Autodesk Fusion 360 part; units mm, degrees
(part 3 of 5)
sketch "Sketch1 (2)" plane through (0, 0, 19.05) normal (0, 0, 1) x (-1, 0, 0) in component "spoilboard v12"
  line L0 (-99.06, -2093.1525) -> (-33.02, -2093.1525)
  arc A0 (-33.02, -2133.1525) -> (-33.02, -2093.1525) centre (-33.02, -2113.1525) ccw
  line L1 (-33.02, -2133.1525) -> (-99.06, -2133.1525)
  arc A1 (-99.06, -2093.1525) -> (-99.06, -2133.1525) centre (-99.06, -2113.1525) ccw
  arc A2 (-461.4333, -1693.1525) -> (-461.4333, -1733.1525) centre (-461.4333, -1713.1525) ccw
  line L2 (-461.4333, -1693.1525) -> (-395.3933, -1693.1525)
  arc A3 (-395.3933, -1733.1525) -> (-395.3933, -1693.1525) centre (-395.3933, -1713.1525) ccw
  line L3 (-395.3933, -1733.1525) -> (-461.4333, -1733.1525)
  line L4 (-99.06, -1913.1525) -> (-33.02, -1913.1525)
  arc A4 (-33.02, -1953.1525) -> (-33.02, -1913.1525) centre (-33.02, -1933.1525) ccw
  line L5 (-33.02, -1953.1525) -> (-99.06, -1953.1525)
  arc A5 (-99.06, -1913.1525) -> (-99.06, -1953.1525) centre (-99.06, -1933.1525) ccw
  line L6 (-99.06, -1293.1525) -> (-33.02, -1293.1525)
  arc A6 (-33.02, -1333.1525) -> (-33.02, -1293.1525) centre (-33.02, -1313.1525) ccw
  line L7 (-33.02, -1333.1525) -> (-99.06, -1333.1525)
  arc A7 (-99.06, -1293.1525) -> (-99.06, -1333.1525) centre (-99.06, -1313.1525) ccw
  arc A8 (-642.62, -2093.1525) -> (-642.62, -2133.1525) centre (-642.62, -2113.1525) ccw
  line L8 (-642.62, -2093.1525) -> (-576.58, -2093.1525)
  arc A9 (-576.58, -2133.1525) -> (-576.58, -2093.1525) centre (-576.58, -2113.1525) ccw
  line L9 (-576.58, -2133.1525) -> (-642.62, -2133.1525)
  arc A10 (-642.62, -2313.1525) -> (-642.62, -2353.1525) centre (-642.62, -2333.1525) ccw
  line L10 (-642.62, -2313.1525) -> (-576.58, -2313.1525)
  arc A11 (-576.58, -2353.1525) -> (-576.58, -2313.1525) centre (-576.58, -2333.1525) ccw
  line L11 (-576.58, -2353.1525) -> (-642.62, -2353.1525)
  arc A12 (-642.62, -1693.1525) -> (-642.62, -1733.1525) centre (-642.62, -1713.1525) ccw
  line L12 (-642.62, -1693.1525) -> (-576.58, -1693.1525)
  arc A13 (-576.58, -1733.1525) -> (-576.58, -1693.1525) centre (-576.58, -1713.1525) ccw
  line L13 (-576.58, -1733.1525) -> (-642.62, -1733.1525)
  arc A14 (-642.62, -1913.1525) -> (-642.62, -1953.1525) centre (-642.62, -1933.1525) ccw
  line L14 (-642.62, -1913.1525) -> (-576.58, -1913.1525)
  arc A15 (-576.58, -1953.1525) -> (-576.58, -1913.1525) centre (-576.58, -1933.1525) ccw
  line L15 (-576.58, -1953.1525) -> (-642.62, -1953.1525)
  arc A16 (-642.62, -1293.1525) -> (-642.62, -1333.1525) centre (-642.62, -1313.1525) ccw
  line L16 (-642.62, -1293.1525) -> (-576.58, -1293.1525)
  arc A17 (-576.58, -1333.1525) -> (-576.58, -1293.1525) centre (-576.58, -1313.1525) ccw
  line L17 (-576.58, -1333.1525) -> (-642.62, -1333.1525)
  arc A18 (-642.62, -1513.1525) -> (-642.62, -1553.1525) centre (-642.62, -1533.1525) ccw
  line L18 (-642.62, -1513.1525) -> (-576.58, -1513.1525)
  arc A19 (-576.58, -1553.1525) -> (-576.58, -1513.1525) centre (-576.58, -1533.1525) ccw
  line L19 (-576.58, -1553.1525) -> (-642.62, -1553.1525)
  line L20 (-33.02, -133.1525) -> (-99.06, -133.1525)
  arc A20 (-99.06, -93.1525) -> (-99.06, -133.1525) centre (-99.06, -113.1525) ccw
  line L21 (-99.06, -93.1525) -> (-33.02, -93.1525)
  arc A21 (-33.02, -133.1525) -> (-33.02, -93.1525) centre (-33.02, -113.1525) ccw
  line L22 (-214.2067, -353.1525) -> (-280.2467, -353.1525)
  arc A22 (-280.2467, -313.1525) -> (-280.2467, -353.1525) centre (-280.2467, -333.1525) ccw
  line L23 (-280.2467, -313.1525) -> (-214.2067, -313.1525)
  arc A23 (-214.2067, -353.1525) -> (-214.2067, -313.1525) centre (-214.2067, -333.1525) ccw
  arc A24 (-461.4333, -713.1525) -> (-461.4333, -753.1525) centre (-461.4333, -733.1525) ccw
  line L24 (-461.4333, -713.1525) -> (-395.3933, -713.1525)
  arc A25 (-395.3933, -753.1525) -> (-395.3933, -713.1525) centre (-395.3933, -733.1525) ccw
  line L25 (-395.3933, -753.1525) -> (-461.4333, -753.1525)
  arc A26 (-280.2467, -1113.1525) -> (-280.2467, -1153.1525) centre (-280.2467, -1133.1525) ccw
  line L26 (-280.2467, -1113.1525) -> (-214.2067, -1113.1525)
  arc A27 (-214.2067, -1153.1525) -> (-214.2067, -1113.1525) centre (-214.2067, -1133.1525) ccw
  line L27 (-214.2067, -1153.1525) -> (-280.2467, -1153.1525)
  line L28 (-280.2467, -893.1525) -> (-214.2067, -893.1525)
  arc A28 (-214.2067, -933.1525) -> (-214.2067, -893.1525) centre (-214.2067, -913.1525) ccw
  line L29 (-214.2067, -933.1525) -> (-280.2467, -933.1525)
  arc A29 (-280.2467, -893.1525) -> (-280.2467, -933.1525) centre (-280.2467, -913.1525) ccw
  line L30 (-1120.14, -133.1525) -> (-1186.18, -133.1525)
  arc A30 (-1186.18, -93.1525) -> (-1186.18, -133.1525) centre (-1186.18, -113.1525) ccw
  line L31 (-1186.18, -93.1525) -> (-1120.14, -93.1525)
  arc A31 (-1120.14, -133.1525) -> (-1120.14, -93.1525) centre (-1120.14, -113.1525) ccw
  line L32 (-1120.14, -353.1525) -> (-1186.18, -353.1525)
  arc A32 (-1186.18, -313.1525) -> (-1186.18, -353.1525) centre (-1186.18, -333.1525) ccw
  line L33 (-1186.18, -313.1525) -> (-1120.14, -313.1525)
  arc A33 (-1120.14, -353.1525) -> (-1120.14, -313.1525) centre (-1120.14, -333.1525) ccw
  arc A34 (-642.62, -713.1525) -> (-642.62, -753.1525) centre (-642.62, -733.1525) ccw
  line L34 (-642.62, -713.1525) -> (-576.58, -713.1525)
  arc A35 (-576.58, -753.1525) -> (-576.58, -713.1525) centre (-576.58, -733.1525) ccw
  line L35 (-576.58, -753.1525) -> (-642.62, -753.1525)
  arc A36 (-642.62, -493.1525) -> (-642.62, -533.1525) centre (-642.62, -513.1525) ccw
  line L36 (-642.62, -493.1525) -> (-576.58, -493.1525)
  arc A37 (-576.58, -533.1525) -> (-576.58, -493.1525) centre (-576.58, -513.1525) ccw
  line L37 (-576.58, -533.1525) -> (-642.62, -533.1525)
  arc A38 (-642.62, -1113.1525) -> (-642.62, -1153.1525) centre (-642.62, -1133.1525) ccw
  line L38 (-642.62, -1113.1525) -> (-576.58, -1113.1525)
  arc A39 (-576.58, -1153.1525) -> (-576.58, -1113.1525) centre (-576.58, -1133.1525) ccw
  line L39 (-576.58, -1153.1525) -> (-642.62, -1153.1525)
  arc A40 (-642.62, -893.1525) -> (-642.62, -933.1525) centre (-642.62, -913.1525) ccw
  line L40 (-642.62, -893.1525) -> (-576.58, -893.1525)
  arc A41 (-576.58, -933.1525) -> (-576.58, -893.1525) centre (-576.58, -913.1525) ccw
  line L41 (-576.58, -933.1525) -> (-642.62, -933.1525)
  line L42 (-757.7667, -933.1525) -> (-823.8067, -933.1525)
  arc A42 (-823.8067, -893.1525) -> (-823.8067, -933.1525) centre (-823.8067, -913.1525) ccw
  line L43 (-823.8067, -893.1525) -> (-757.7667, -893.1525)
  arc A43 (-757.7667, -933.1525) -> (-757.7667, -893.1525) centre (-757.7667, -913.1525) ccw
  line L44 (-757.7667, -1153.1525) -> (-823.8067, -1153.1525)
  arc A44 (-823.8067, -1113.1525) -> (-823.8067, -1153.1525) centre (-823.8067, -1133.1525) ccw
  line L45 (-823.8067, -1113.1525) -> (-757.7667, -1113.1525)
  arc A45 (-757.7667, -1153.1525) -> (-757.7667, -1113.1525) centre (-757.7667, -1133.1525) ccw
  line L46 (-757.7667, -533.1525) -> (-823.8067, -533.1525)
  arc A46 (-823.8067, -493.1525) -> (-823.8067, -533.1525) centre (-823.8067, -513.1525) ccw
  line L47 (-823.8067, -493.1525) -> (-757.7667, -493.1525)
  arc A47 (-757.7667, -533.1525) -> (-757.7667, -493.1525) centre (-757.7667, -513.1525) ccw
  line L48 (-757.7667, -753.1525) -> (-823.8067, -753.1525)
  arc A48 (-823.8067, -713.1525) -> (-823.8067, -753.1525) centre (-823.8067, -733.1525) ccw
  line L49 (-823.8067, -713.1525) -> (-757.7667, -713.1525)
  arc A49 (-757.7667, -753.1525) -> (-757.7667, -713.1525) centre (-757.7667, -733.1525) ccw
  line L50 (-938.9533, -353.1525) -> (-1004.9933, -353.1525)
  arc A50 (-1004.9933, -313.1525) -> (-1004.9933, -353.1525) centre (-1004.9933, -333.1525) ccw
  line L51 (-1004.9933, -313.1525) -> (-938.9533, -313.1525)
  arc A51 (-938.9533, -353.1525) -> (-938.9533, -313.1525) centre (-938.9533, -333.1525) ccw
  line L52 (-938.9533, -133.1525) -> (-1004.9933, -133.1525)
  arc A52 (-1004.9933, -93.1525) -> (-1004.9933, -133.1525) centre (-1004.9933, -113.1525) ccw
  line L53 (-1004.9933, -93.1525) -> (-938.9533, -93.1525)
  arc A53 (-938.9533, -133.1525) -> (-938.9533, -93.1525) centre (-938.9533, -113.1525) ccw
  line L54 (-99.06, -893.1525) -> (-33.02, -893.1525)
  arc A54 (-33.02, -933.1525) -> (-33.02, -893.1525) centre (-33.02, -913.1525) ccw
  line L55 (-33.02, -933.1525) -> (-99.06, -933.1525)
  arc A55 (-99.06, -893.1525) -> (-99.06, -933.1525) centre (-99.06, -913.1525) ccw
  arc A56 (-461.4333, -493.1525) -> (-461.4333, -533.1525) centre (-461.4333, -513.1525) ccw
  line L56 (-461.4333, -493.1525) -> (-395.3933, -493.1525)
  arc A57 (-395.3933, -533.1525) -> (-395.3933, -493.1525) centre (-395.3933, -513.1525) ccw
  line L57 (-395.3933, -533.1525) -> (-461.4333, -533.1525)
  line L58 (-99.06, -713.1525) -> (-33.02, -713.1525)
  arc A58 (-33.02, -753.1525) -> (-33.02, -713.1525) centre (-33.02, -733.1525) ccw
  line L59 (-33.02, -753.1525) -> (-99.06, -753.1525)
  arc A59 (-99.06, -713.1525) -> (-99.06, -753.1525) centre (-99.06, -733.1525) ccw
  line L60 (-33.02, -353.1525) -> (-99.06, -353.1525)
  arc A60 (-99.06, -313.1525) -> (-99.06, -353.1525) centre (-99.06, -333.1525) ccw
  line L61 (-99.06, -313.1525) -> (-33.02, -313.1525)
  arc A61 (-33.02, -353.1525) -> (-33.02, -313.1525) centre (-33.02, -333.1525) ccw
  line L62 (-1186.18, -1513.1525) -> (-1120.14, -1513.1525)
  arc A62 (-1120.14, -1553.1525) -> (-1120.14, -1513.1525) centre (-1120.14, -1533.1525) ccw
  line L63 (-1120.14, -1553.1525) -> (-1186.18, -1553.1525)
  arc A63 (-1186.18, -1513.1525) -> (-1186.18, -1553.1525) centre (-1186.18, -1533.1525) ccw
  line L64 (-1120.14, -1333.1525) -> (-1186.18, -1333.1525)
  arc A64 (-1186.18, -1293.1525) -> (-1186.18, -1333.1525) centre (-1186.18, -1313.1525) ccw
  line L65 (-1186.18, -1293.1525) -> (-1120.14, -1293.1525)
  arc A65 (-1120.14, -1333.1525) -> (-1120.14, -1293.1525) centre (-1120.14, -1313.1525) ccw
  line L66 (-1186.18, -1913.1525) -> (-1120.14, -1913.1525)
  arc A66 (-1120.14, -1953.1525) -> (-1120.14, -1913.1525) centre (-1120.14, -1933.1525) ccw
  line L67 (-1120.14, -1953.1525) -> (-1186.18, -1953.1525)
  arc A67 (-1186.18, -1913.1525) -> (-1186.18, -1953.1525) centre (-1186.18, -1933.1525) ccw
  line L68 (-1120.14, -1733.1525) -> (-1186.18, -1733.1525)
  arc A68 (-1186.18, -1693.1525) -> (-1186.18, -1733.1525) centre (-1186.18, -1713.1525) ccw
  line L69 (-1186.18, -1693.1525) -> (-1120.14, -1693.1525)
  arc A69 (-1120.14, -1733.1525) -> (-1120.14, -1693.1525) centre (-1120.14, -1713.1525) ccw
  line L70 (-1186.18, -2313.1525) -> (-1120.14, -2313.1525)
  arc A70 (-1120.14, -2353.1525) -> (-1120.14, -2313.1525) centre (-1120.14, -2333.1525) ccw
  line L71 (-1120.14, -2353.1525) -> (-1186.18, -2353.1525)
  arc A71 (-1186.18, -2313.1525) -> (-1186.18, -2353.1525) centre (-1186.18, -2333.1525) ccw
  line L72 (-1120.14, -2133.1525) -> (-1186.18, -2133.1525)
  arc A72 (-1186.18, -2093.1525) -> (-1186.18, -2133.1525) centre (-1186.18, -2113.1525) ccw
  line L73 (-1186.18, -2093.1525) -> (-1120.14, -2093.1525)
  arc A73 (-1120.14, -2133.1525) -> (-1120.14, -2093.1525) centre (-1120.14, -2113.1525) ccw
  arc A74 (-280.2467, -1513.1525) -> (-280.2467, -1553.1525) centre (-280.2467, -1533.1525) ccw
  line L74 (-280.2467, -1513.1525) -> (-214.2067, -1513.1525)
  arc A75 (-214.2067, -1553.1525) -> (-214.2067, -1513.1525) centre (-214.2067, -1533.1525) ccw
  line L75 (-214.2067, -1553.1525) -> (-280.2467, -1553.1525)
  line L76 (-280.2467, -1293.1525) -> (-214.2067, -1293.1525)
  arc A76 (-214.2067, -1333.1525) -> (-214.2067, -1293.1525) centre (-214.2067, -1313.1525) ccw
  line L77 (-214.2067, -1333.1525) -> (-280.2467, -1333.1525)
  arc A77 (-280.2467, -1293.1525) -> (-280.2467, -1333.1525) centre (-280.2467, -1313.1525) ccw
  arc A78 (-461.4333, -1913.1525) -> (-461.4333, -1953.1525) centre (-461.4333, -1933.1525) ccw
  line L78 (-461.4333, -1913.1525) -> (-395.3933, -1913.1525)
  arc A79 (-395.3933, -1953.1525) -> (-395.3933, -1913.1525) centre (-395.3933, -1933.1525) ccw
  line L79 (-395.3933, -1953.1525) -> (-461.4333, -1953.1525)
  arc A80 (-280.2467, -2313.1525) -> (-280.2467, -2353.1525) centre (-280.2467, -2333.1525) ccw
  line L80 (-280.2467, -2313.1525) -> (-214.2067, -2313.1525)
  arc A81 (-214.2067, -2353.1525) -> (-214.2067, -2313.1525) centre (-214.2067, -2333.1525) ccw
  line L81 (-214.2067, -2353.1525) -> (-280.2467, -2353.1525)
  line L82 (-280.2467, -2093.1525) -> (-214.2067, -2093.1525)
  arc A82 (-214.2067, -2133.1525) -> (-214.2067, -2093.1525) centre (-214.2067, -2113.1525) ccw
  line L83 (-214.2067, -2133.1525) -> (-280.2467, -2133.1525)
  arc A83 (-280.2467, -2093.1525) -> (-280.2467, -2133.1525) centre (-280.2467, -2113.1525) ccw
  arc A84 (-461.4333, -2313.1525) -> (-461.4333, -2353.1525) centre (-461.4333, -2333.1525) ccw
  line L84 (-461.4333, -2313.1525) -> (-395.3933, -2313.1525)
  arc A85 (-395.3933, -2353.1525) -> (-395.3933, -2313.1525) centre (-395.3933, -2333.1525) ccw
  line L85 (-395.3933, -2353.1525) -> (-461.4333, -2353.1525)
  line L86 (-280.2467, -1693.1525) -> (-214.2067, -1693.1525)
  arc A86 (-214.2067, -1733.1525) -> (-214.2067, -1693.1525) centre (-214.2067, -1713.1525) ccw
  line L87 (-214.2067, -1733.1525) -> (-280.2467, -1733.1525)
  arc A87 (-280.2467, -1693.1525) -> (-280.2467, -1733.1525) centre (-280.2467, -1713.1525) ccw
  arc A88 (-280.2467, -1913.1525) -> (-280.2467, -1953.1525) centre (-280.2467, -1933.1525) ccw
  line L88 (-280.2467, -1913.1525) -> (-214.2067, -1913.1525)
  arc A89 (-214.2067, -1953.1525) -> (-214.2067, -1913.1525) centre (-214.2067, -1933.1525) ccw
  line L89 (-214.2067, -1953.1525) -> (-280.2467, -1953.1525)
  arc A90 (-461.4333, -1513.1525) -> (-461.4333, -1553.1525) centre (-461.4333, -1533.1525) ccw
  line L90 (-461.4333, -1513.1525) -> (-395.3933, -1513.1525)
  arc A91 (-395.3933, -1553.1525) -> (-395.3933, -1513.1525) centre (-395.3933, -1533.1525) ccw
  line L91 (-395.3933, -1553.1525) -> (-461.4333, -1553.1525)
  line L92 (-757.7667, -2133.1525) -> (-823.8067, -2133.1525)
  arc A92 (-823.8067, -2093.1525) -> (-823.8067, -2133.1525) centre (-823.8067, -2113.1525) ccw
  line L93 (-823.8067, -2093.1525) -> (-757.7667, -2093.1525)
  arc A93 (-757.7667, -2133.1525) -> (-757.7667, -2093.1525) centre (-757.7667, -2113.1525) ccw
  line L94 (-757.7667, -2353.1525) -> (-823.8067, -2353.1525)
  arc A94 (-823.8067, -2313.1525) -> (-823.8067, -2353.1525) centre (-823.8067, -2333.1525) ccw
  line L95 (-823.8067, -2313.1525) -> (-757.7667, -2313.1525)
  arc A95 (-757.7667, -2353.1525) -> (-757.7667, -2313.1525) centre (-757.7667, -2333.1525) ccw
  line L96 (-757.7667, -1733.1525) -> (-823.8067, -1733.1525)
  arc A96 (-823.8067, -1693.1525) -> (-823.8067, -1733.1525) centre (-823.8067, -1713.1525) ccw
  line L97 (-823.8067, -1693.1525) -> (-757.7667, -1693.1525)
  arc A97 (-757.7667, -1733.1525) -> (-757.7667, -1693.1525) centre (-757.7667, -1713.1525) ccw
  line L98 (-757.7667, -1953.1525) -> (-823.8067, -1953.1525)
  arc A98 (-823.8067, -1913.1525) -> (-823.8067, -1953.1525) centre (-823.8067, -1933.1525) ccw
  line L99 (-823.8067, -1913.1525) -> (-757.7667, -1913.1525)
  arc A99 (-757.7667, -1953.1525) -> (-757.7667, -1913.1525) centre (-757.7667, -1933.1525) ccw
  line L100 (-757.7667, -1333.1525) -> (-823.8067, -1333.1525)
  arc A100 (-823.8067, -1293.1525) -> (-823.8067, -1333.1525) centre (-823.8067, -1313.1525) ccw
  line L101 (-823.8067, -1293.1525) -> (-757.7667, -1293.1525)
  arc A101 (-757.7667, -1333.1525) -> (-757.7667, -1293.1525) centre (-757.7667, -1313.1525) ccw
  line L102 (-757.7667, -1553.1525) -> (-823.8067, -1553.1525)
  arc A102 (-823.8067, -1513.1525) -> (-823.8067, -1553.1525) centre (-823.8067, -1533.1525) ccw
  line L103 (-823.8067, -1513.1525) -> (-757.7667, -1513.1525)
  arc A103 (-757.7667, -1553.1525) -> (-757.7667, -1513.1525) centre (-757.7667, -1533.1525) ccw
  line L104 (-214.2067, -133.1525) -> (-280.2467, -133.1525)
  arc A104 (-280.2467, -93.1525) -> (-280.2467, -133.1525) centre (-280.2467, -113.1525) ccw
  line L105 (-280.2467, -93.1525) -> (-214.2067, -93.1525)
  arc A105 (-214.2067, -133.1525) -> (-214.2067, -93.1525) centre (-214.2067, -113.1525) ccw
  line L106 (-395.3933, -353.1525) -> (-461.4333, -353.1525)
  arc A106 (-461.4333, -313.1525) -> (-461.4333, -353.1525) centre (-461.4333, -333.1525) ccw
  line L107 (-461.4333, -313.1525) -> (-395.3933, -313.1525)
  arc A107 (-395.3933, -353.1525) -> (-395.3933, -313.1525) centre (-395.3933, -333.1525) ccw
  line L108 (-99.06, -493.1525) -> (-33.02, -493.1525)
  arc A108 (-33.02, -533.1525) -> (-33.02, -493.1525) centre (-33.02, -513.1525) ccw
  line L109 (-33.02, -533.1525) -> (-99.06, -533.1525)
  arc A109 (-99.06, -493.1525) -> (-99.06, -533.1525) centre (-99.06, -513.1525) ccw
  line L110 (-99.06, -1113.1525) -> (-33.02, -1113.1525)
  arc A110 (-33.02, -1153.1525) -> (-33.02, -1113.1525) centre (-33.02, -1133.1525) ccw
  line L111 (-33.02, -1153.1525) -> (-99.06, -1153.1525)
  arc A111 (-99.06, -1113.1525) -> (-99.06, -1153.1525) centre (-99.06, -1133.1525) ccw
  arc A112 (-461.4333, -893.1525) -> (-461.4333, -933.1525) centre (-461.4333, -913.1525) ccw
  line L112 (-461.4333, -893.1525) -> (-395.3933, -893.1525)
  arc A113 (-395.3933, -933.1525) -> (-395.3933, -893.1525) centre (-395.3933, -913.1525) ccw
  line L113 (-395.3933, -933.1525) -> (-461.4333, -933.1525)
  line L114 (-576.58, -353.1525) -> (-642.62, -353.1525)
  arc A114 (-642.62, -313.1525) -> (-642.62, -353.1525) centre (-642.62, -333.1525) ccw
  line L115 (-642.62, -313.1525) -> (-576.58, -313.1525)
  arc A115 (-576.58, -353.1525) -> (-576.58, -313.1525) centre (-576.58, -333.1525) ccw
  line L116 (-1186.18, -713.1525) -> (-1120.14, -713.1525)
  arc A116 (-1120.14, -753.1525) -> (-1120.14, -713.1525) centre (-1120.14, -733.1525) ccw
  line L117 (-1120.14, -753.1525) -> (-1186.18, -753.1525)
  arc A117 (-1186.18, -713.1525) -> (-1186.18, -753.1525) centre (-1186.18, -733.1525) ccw
  line L118 (-1120.14, -533.1525) -> (-1186.18, -533.1525)
  arc A118 (-1186.18, -493.1525) -> (-1186.18, -533.1525) centre (-1186.18, -513.1525) ccw
  line L119 (-1186.18, -493.1525) -> (-1120.14, -493.1525)
  arc A119 (-1120.14, -533.1525) -> (-1120.14, -493.1525) centre (-1120.14, -513.1525) ccw
  line L120 (-1186.18, -1113.1525) -> (-1120.14, -1113.1525)
  arc A120 (-1120.14, -1153.1525) -> (-1120.14, -1113.1525) centre (-1120.14, -1133.1525) ccw
  line L121 (-1120.14, -1153.1525) -> (-1186.18, -1153.1525)
  arc A121 (-1186.18, -1113.1525) -> (-1186.18, -1153.1525) centre (-1186.18, -1133.1525) ccw
  line L122 (-1120.14, -933.1525) -> (-1186.18, -933.1525)
  arc A122 (-1186.18, -893.1525) -> (-1186.18, -933.1525) centre (-1186.18, -913.1525) ccw
  line L123 (-1186.18, -893.1525) -> (-1120.14, -893.1525)
  arc A123 (-1120.14, -933.1525) -> (-1120.14, -893.1525) centre (-1120.14, -913.1525) ccw
  line L124 (-576.58, -133.1525) -> (-642.62, -133.1525)
  arc A124 (-642.62, -93.1525) -> (-642.62, -133.1525) centre (-642.62, -113.1525) ccw
  line L125 (-642.62, -93.1525) -> (-576.58, -93.1525)
  arc A125 (-576.58, -133.1525) -> (-576.58, -93.1525) centre (-576.58, -113.1525) ccw
  line L126 (-938.9533, -933.1525) -> (-1004.9933, -933.1525)
  arc A126 (-1004.9933, -893.1525) -> (-1004.9933, -933.1525) centre (-1004.9933, -913.1525) ccw
  line L127 (-1004.9933, -893.1525) -> (-938.9533, -893.1525)
  arc A127 (-938.9533, -933.1525) -> (-938.9533, -893.1525) centre (-938.9533, -913.1525) ccw
  arc A128 (-1004.9933, -1113.1525) -> (-1004.9933, -1153.1525) centre (-1004.9933, -1133.1525) ccw
  line L128 (-1004.9933, -1113.1525) -> (-938.9533, -1113.1525)
  arc A129 (-938.9533, -1153.1525) -> (-938.9533, -1113.1525) centre (-938.9533, -1133.1525) ccw
  line L129 (-938.9533, -1153.1525) -> (-1004.9933, -1153.1525)
  line L130 (-938.9533, -533.1525) -> (-1004.9933, -533.1525)
  arc A130 (-1004.9933, -493.1525) -> (-1004.9933, -533.1525) centre (-1004.9933, -513.1525) ccw
  line L131 (-1004.9933, -493.1525) -> (-938.9533, -493.1525)
  arc A131 (-938.9533, -533.1525) -> (-938.9533, -493.1525) centre (-938.9533, -513.1525) ccw
  arc A132 (-1004.9933, -713.1525) -> (-1004.9933, -753.1525) centre (-1004.9933, -733.1525) ccw
  line L132 (-1004.9933, -713.1525) -> (-938.9533, -713.1525)
  arc A133 (-938.9533, -753.1525) -> (-938.9533, -713.1525) centre (-938.9533, -733.1525) ccw
  line L133 (-938.9533, -753.1525) -> (-1004.9933, -753.1525)
  line L134 (-757.7667, -353.1525) -> (-823.8067, -353.1525)
  arc A134 (-823.8067, -313.1525) -> (-823.8067, -353.1525) centre (-823.8067, -333.1525) ccw
  line L135 (-823.8067, -313.1525) -> (-757.7667, -313.1525)
  arc A135 (-757.7667, -353.1525) -> (-757.7667, -313.1525) centre (-757.7667, -333.1525) ccw
  line L136 (-757.7667, -133.1525) -> (-823.8067, -133.1525)
  arc A136 (-823.8067, -93.1525) -> (-823.8067, -133.1525) centre (-823.8067, -113.1525) ccw
  line L137 (-823.8067, -93.1525) -> (-757.7667, -93.1525)
  arc A137 (-757.7667, -133.1525) -> (-757.7667, -93.1525) centre (-757.7667, -113.1525) ccw
  arc A138 (-461.4333, -1113.1525) -> (-461.4333, -1153.1525) centre (-461.4333, -1133.1525) ccw
  line L138 (-461.4333, -1113.1525) -> (-395.3933, -1113.1525)
  arc A139 (-395.3933, -1153.1525) -> (-395.3933, -1113.1525) centre (-395.3933, -1133.1525) ccw
  line L139 (-395.3933, -1153.1525) -> (-461.4333, -1153.1525)
  line L140 (-280.2467, -493.1525) -> (-214.2067, -493.1525)
  arc A140 (-214.2067, -533.1525) -> (-214.2067, -493.1525) centre (-214.2067, -513.1525) ccw
  line L141 (-214.2067, -533.1525) -> (-280.2467, -533.1525)
  arc A141 (-280.2467, -493.1525) -> (-280.2467, -533.1525) centre (-280.2467, -513.1525) ccw
  arc A142 (-280.2467, -713.1525) -> (-280.2467, -753.1525) centre (-280.2467, -733.1525) ccw
  line L142 (-280.2467, -713.1525) -> (-214.2067, -713.1525)
  arc A143 (-214.2067, -753.1525) -> (-214.2067, -713.1525) centre (-214.2067, -733.1525) ccw
  line L143 (-214.2067, -753.1525) -> (-280.2467, -753.1525)
  line L144 (-395.3933, -133.1525) -> (-461.4333, -133.1525)
  arc A144 (-461.4333, -93.1525) -> (-461.4333, -133.1525) centre (-461.4333, -113.1525) ccw
  line L145 (-461.4333, -93.1525) -> (-395.3933, -93.1525)
  arc A145 (-395.3933, -133.1525) -> (-395.3933, -93.1525) centre (-395.3933, -113.1525) ccw
  arc A146 (-1004.9933, -1513.1525) -> (-1004.9933, -1553.1525) centre (-1004.9933, -1533.1525) ccw
  line L146 (-1004.9933, -1513.1525) -> (-938.9533, -1513.1525)
  arc A147 (-938.9533, -1553.1525) -> (-938.9533, -1513.1525) centre (-938.9533, -1533.1525) ccw
  line L147 (-938.9533, -1553.1525) -> (-1004.9933, -1553.1525)
  line L148 (-938.9533, -1333.1525) -> (-1004.9933, -1333.1525)
  arc A148 (-1004.9933, -1293.1525) -> (-1004.9933, -1333.1525) centre (-1004.9933, -1313.1525) ccw
  line L149 (-1004.9933, -1293.1525) -> (-938.9533, -1293.1525)
  arc A149 (-938.9533, -1333.1525) -> (-938.9533, -1293.1525) centre (-938.9533, -1313.1525) ccw
  arc A150 (-1004.9933, -1913.1525) -> (-1004.9933, -1953.1525) centre (-1004.9933, -1933.1525) ccw
  line L150 (-1004.9933, -1913.1525) -> (-938.9533, -1913.1525)
  arc A151 (-938.9533, -1953.1525) -> (-938.9533, -1913.1525) centre (-938.9533, -1933.1525) ccw
  line L151 (-938.9533, -1953.1525) -> (-1004.9933, -1953.1525)
  line L152 (-938.9533, -1733.1525) -> (-1004.9933, -1733.1525)
  arc A152 (-1004.9933, -1693.1525) -> (-1004.9933, -1733.1525) centre (-1004.9933, -1713.1525) ccw
  line L153 (-1004.9933, -1693.1525) -> (-938.9533, -1693.1525)
  arc A153 (-938.9533, -1733.1525) -> (-938.9533, -1693.1525) centre (-938.9533, -1713.1525) ccw
  arc A154 (-1004.9933, -2313.1525) -> (-1004.9933, -2353.1525) centre (-1004.9933, -2333.1525) ccw
  line L154 (-1004.9933, -2313.1525) -> (-938.9533, -2313.1525)
  arc A155 (-938.9533, -2353.1525) -> (-938.9533, -2313.1525) centre (-938.9533, -2333.1525) ccw
  line L155 (-938.9533, -2353.1525) -> (-1004.9933, -2353.1525)
  line L156 (-938.9533, -2133.1525) -> (-1004.9933, -2133.1525)
  arc A156 (-1004.9933, -2093.1525) -> (-1004.9933, -2133.1525) centre (-1004.9933, -2113.1525) ccw
  line L157 (-1004.9933, -2093.1525) -> (-938.9533, -2093.1525)
  arc A157 (-938.9533, -2133.1525) -> (-938.9533, -2093.1525) centre (-938.9533, -2113.1525) ccw
  line L158 (-99.06, -1513.1525) -> (-33.02, -1513.1525)
  arc A158 (-33.02, -1553.1525) -> (-33.02, -1513.1525) centre (-33.02, -1533.1525) ccw
  line L159 (-33.02, -1553.1525) -> (-99.06, -1553.1525)
  arc A159 (-99.06, -1513.1525) -> (-99.06, -1553.1525) centre (-99.06, -1533.1525) ccw
  arc A160 (-461.4333, -1293.1525) -> (-461.4333, -1333.1525) centre (-461.4333, -1313.1525) ccw
  line L160 (-461.4333, -1293.1525) -> (-395.3933, -1293.1525)
  arc A161 (-395.3933, -1333.1525) -> (-395.3933, -1293.1525) centre (-395.3933, -1313.1525) ccw
  line L161 (-395.3933, -1333.1525) -> (-461.4333, -1333.1525)
  line L162 (-99.06, -1693.1525) -> (-33.02, -1693.1525)
  arc A162 (-33.02, -1733.1525) -> (-33.02, -1693.1525) centre (-33.02, -1713.1525) ccw
  line L163 (-33.02, -1733.1525) -> (-99.06, -1733.1525)
  arc A163 (-99.06, -1693.1525) -> (-99.06, -1733.1525) centre (-99.06, -1713.1525) ccw
  line L164 (-99.06, -2313.1525) -> (-33.02, -2313.1525)
  arc A164 (-33.02, -2353.1525) -> (-33.02, -2313.1525) centre (-33.02, -2333.1525) ccw
  line L165 (-33.02, -2353.1525) -> (-99.06, -2353.1525)
  arc A165 (-99.06, -2313.1525) -> (-99.06, -2353.1525) centre (-99.06, -2333.1525) ccw
  arc A166 (-461.4333, -2093.1525) -> (-461.4333, -2133.1525) centre (-461.4333, -2113.1525) ccw
  line L166 (-461.4333, -2093.1525) -> (-395.3933, -2093.1525)
  arc A167 (-395.3933, -2133.1525) -> (-395.3933, -2093.1525) centre (-395.3933, -2113.1525) ccw
  line L167 (-395.3933, -2133.1525) -> (-461.4333, -2133.1525)
  circle A168 centre (-34.29, -2020) radius 17.145
  circle A169 centre (-321.945, -2020) radius 17.145
  circle A170 centre (-609.6, -2020) radius 17.145
  circle A171 centre (-321.945, -420) radius 17.145
  circle A172 centre (-897.255, -2020) radius 17.145
  circle A173 centre (-1184.91, -2020) radius 17.145
  circle A174 centre (-34.29, -420) radius 17.145
  circle A175 centre (-34.29, -2420) radius 17.145
  circle A176 centre (-1184.91, -20) radius 17.145
  circle A177 centre (-321.945, -2420) radius 17.145
  circle A178 centre (-609.6, -2420) radius 17.145
  circle A179 centre (-897.255, -20) radius 17.145
  circle A180 centre (-897.255, -2420) radius 17.145
  circle A181 centre (-321.945, -1220) radius 17.145
  circle A182 centre (-34.29, -1220) radius 17.145
  circle A183 centre (-1184.91, -820) radius 17.145
  circle A184 centre (-897.255, -820) radius 17.145
  circle A185 centre (-609.6, -820) radius 17.145
  circle A186 centre (-34.29, -20) radius 17.145
  circle A187 centre (-1184.91, -2420) radius 17.145
  circle A188 centre (-609.6, -20) radius 17.145
  circle A189 centre (-321.945, -20) radius 17.145
  circle A190 centre (-609.6, -1620) radius 17.145
  circle A191 centre (-897.255, -1620) radius 17.145
  circle A192 centre (-321.945, -1620) radius 17.145
  circle A193 centre (-34.29, -1620) radius 17.145
  circle A194 centre (-34.29, -820) radius 17.145
  circle A195 centre (-1184.91, -420) radius 17.145
  circle A196 centre (-1184.91, -1220) radius 17.145
  circle A197 centre (-897.255, -1220) radius 17.145
  circle A198 centre (-321.945, -820) radius 17.145
  circle A199 centre (-609.6, -1220) radius 17.145
  circle A200 centre (-609.6, -420) radius 17.145
  circle A201 centre (-897.255, -420) radius 17.145
  circle A202 centre (-1184.91, -1620) radius 17.145
  line L168 (0, 0) -> (-1219.2, 0)
  line L169 (-1219.2, 0) -> (-1219.2, -2463.8)
  line L170 (-1219.2, -2463.8) -> (0, -2463.8)
  line L171 (0, -2463.8) -> (0, 0)
  line L172 (90.1264, -25.4) -> (-1609.7775, -25.4) construction
  circle A203 centre (-250.825, -22.225) radius 3.175
  line L173 (-171.45, -2550) -> (-171.45, 84.677) construction
  line L174 (-254, -71.5891) -> (-254, 71.5891) construction
  line L175 (-1016, -114.2016) -> (-1016, 104.2016) construction
  circle A204 centre (-1012.825, -22.225) radius 3.175
  circle A205 centre (-171.45, -165.1) radius 9.525
  line L176 (-666.0507, -2247.1575) -> (-731.5763, -2247.1637)
  arc A206 (-731.5761, -2207.1637) -> (-731.5763, -2247.1637) centre (-731.5762, -2227.1637) ccw
  line L177 (-731.5761, -2207.1637) -> (-665.5361, -2207.1642)
  arc A207 (-666.0507, -2247.1575) -> (-665.5361, -2207.1642) centre (-666.0526, -2227.1575) ccw
  line L178 (-1036.0507, -1847.1575) -> (-1101.5763, -1847.1637)
  arc A208 (-1101.5761, -1807.1637) -> (-1101.5763, -1847.1637) centre (-1101.5762, -1827.1637) ccw
  line L179 (-1101.5761, -1807.1637) -> (-1035.5361, -1807.1642)
  arc A209 (-1036.0507, -1847.1575) -> (-1035.5361, -1807.1642) centre (-1036.0526, -1827.1575) ccw
  line L180 (-368.6639, -1807.1642) -> (-302.6239, -1807.1637)
  arc A210 (-302.6237, -1847.1637) -> (-302.6239, -1807.1637) centre (-302.6238, -1827.1637) ccw
  line L181 (-302.6237, -1847.1637) -> (-368.1493, -1847.1575)
  arc A211 (-368.6639, -1807.1642) -> (-368.1493, -1847.1575) centre (-368.1474, -1827.1575) ccw
  line L182 (-666.0507, -1447.1575) -> (-731.5763, -1447.1637)
  arc A212 (-731.5761, -1407.1637) -> (-731.5763, -1447.1637) centre (-731.5762, -1427.1637) ccw
  line L183 (-731.5761, -1407.1637) -> (-665.5361, -1407.1642)
  arc A213 (-666.0507, -1447.1575) -> (-665.5361, -1407.1642) centre (-666.0526, -1427.1575) ccw
  line L184 (-1101.5761, -207.1637) -> (-1035.5361, -207.1642)
  arc A214 (-1036.0507, -247.1575) -> (-1035.5361, -207.1642) centre (-1036.0526, -227.1575) ccw
  line L185 (-1036.0507, -247.1575) -> (-1101.5763, -247.1637)
  arc A215 (-1101.5761, -207.1637) -> (-1101.5763, -247.1637) centre (-1101.5762, -227.1637) ccw
  line L186 (-368.6639, -207.1642) -> (-302.6239, -207.1637)
  arc A216 (-302.6237, -247.1637) -> (-302.6239, -207.1637) centre (-302.6238, -227.1637) ccw
  line L187 (-302.6237, -247.1637) -> (-368.1493, -247.1575)
  arc A217 (-368.6639, -207.1642) -> (-368.1493, -247.1575) centre (-368.1474, -227.1575) ccw
  line L188 (-553.6639, -607.1642) -> (-487.6239, -607.1637)
  arc A218 (-487.6237, -647.1637) -> (-487.6239, -607.1637) centre (-487.6238, -627.1637) ccw
  line L189 (-487.6237, -647.1637) -> (-553.1493, -647.1575)
  arc A219 (-553.6639, -607.1642) -> (-553.1493, -647.1575) centre (-553.1474, -627.1575) ccw
  line L190 (-1036.0507, -1047.1575) -> (-1101.5763, -1047.1637)
  arc A220 (-1101.5761, -1007.1637) -> (-1101.5763, -1047.1637) centre (-1101.5762, -1027.1637) ccw
  line L191 (-1101.5761, -1007.1637) -> (-1035.5361, -1007.1642)
  arc A221 (-1036.0507, -1047.1575) -> (-1035.5361, -1007.1642) centre (-1036.0526, -1027.1575) ccw
  line L192 (-368.6639, -1007.1642) -> (-302.6239, -1007.1637)
  arc A222 (-302.6237, -1047.1637) -> (-302.6239, -1007.1637) centre (-302.6238, -1027.1637) ccw
  line L193 (-302.6237, -1047.1637) -> (-368.1493, -1047.1575)
  arc A223 (-368.6639, -1007.1642) -> (-368.1493, -1047.1575) centre (-368.1474, -1027.1575) ccw
  line L194 (-553.6639, -1007.1642) -> (-487.6239, -1007.1637)
  arc A224 (-487.6237, -1047.1637) -> (-487.6239, -1007.1637) centre (-487.6238, -1027.1637) ccw
  line L195 (-487.6237, -1047.1637) -> (-553.1493, -1047.1575)
  arc A225 (-553.6639, -1007.1642) -> (-553.1493, -1047.1575) centre (-553.1474, -1027.1575) ccw
  line L196 (-1036.0507, -647.1575) -> (-1101.5763, -647.1637)
  arc A226 (-1101.5761, -607.1637) -> (-1101.5763, -647.1637) centre (-1101.5762, -627.1637) ccw
  line L197 (-1101.5761, -607.1637) -> (-1035.5361, -607.1642)
  arc A227 (-1036.0507, -647.1575) -> (-1035.5361, -607.1642) centre (-1036.0526, -627.1575) ccw
  line L198 (-368.6639, -607.1642) -> (-302.6239, -607.1637)
  arc A228 (-302.6237, -647.1637) -> (-302.6239, -607.1637) centre (-302.6238, -627.1637) ccw
  line L199 (-302.6237, -647.1637) -> (-368.1493, -647.1575)
  arc A229 (-368.6639, -607.1642) -> (-368.1493, -647.1575) centre (-368.1474, -627.1575) ccw
  line L200 (-553.6639, -207.1642) -> (-487.6239, -207.1637)
  arc A230 (-487.6237, -247.1637) -> (-487.6239, -207.1637) centre (-487.6238, -227.1637) ccw
  line L201 (-487.6237, -247.1637) -> (-553.1493, -247.1575)
  arc A231 (-553.6639, -207.1642) -> (-553.1493, -247.1575) centre (-553.1474, -227.1575) ccw
  line L202 (-183.6639, -1407.1642) -> (-117.6239, -1407.1637)
  arc A232 (-117.6237, -1447.1637) -> (-117.6239, -1407.1637) centre (-117.6238, -1427.1637) ccw
  line L203 (-117.6237, -1447.1637) -> (-183.1493, -1447.1575)
  arc A233 (-183.6639, -1407.1642) -> (-183.1493, -1447.1575) centre (-183.1474, -1427.1575) ccw
  arc A234 (-916.5761, -1407.1637) -> (-916.5763, -1447.1637) centre (-916.5762, -1427.1637) ccw
  line L204 (-916.5761, -1407.1637) -> (-850.5361, -1407.1642)
  arc A235 (-851.0507, -1447.1575) -> (-850.5361, -1407.1642) centre (-851.0526, -1427.1575) ccw
  line L205 (-851.0507, -1447.1575) -> (-916.5763, -1447.1637)
  line L206 (-553.6639, -1807.1642) -> (-487.6239, -1807.1637)
  arc A236 (-487.6237, -1847.1637) -> (-487.6239, -1807.1637) centre (-487.6238, -1827.1637) ccw
  line L207 (-487.6237, -1847.1637) -> (-553.1493, -1847.1575)
  arc A237 (-553.6639, -1807.1642) -> (-553.1493, -1847.1575) centre (-553.1474, -1827.1575) ccw
  line L208 (-183.6639, -2207.1642) -> (-117.6239, -2207.1637)
  arc A238 (-117.6237, -2247.1637) -> (-117.6239, -2207.1637) centre (-117.6238, -2227.1637) ccw
  line L209 (-117.6237, -2247.1637) -> (-183.1493, -2247.1575)
  arc A239 (-183.6639, -2207.1642) -> (-183.1493, -2247.1575) centre (-183.1474, -2227.1575) ccw
  arc A240 (-916.5761, -2207.1637) -> (-916.5763, -2247.1637) centre (-916.5762, -2227.1637) ccw
  line L210 (-916.5761, -2207.1637) -> (-850.5361, -2207.1642)
  arc A241 (-851.0507, -2247.1575) -> (-850.5361, -2207.1642) centre (-851.0526, -2227.1575) ccw
  line L211 (-851.0507, -2247.1575) -> (-916.5763, -2247.1637)
  line L212 (-553.6639, -2207.1642) -> (-487.6239, -2207.1637)
  arc A242 (-487.6237, -2247.1637) -> (-487.6239, -2207.1637) centre (-487.6238, -2227.1637) ccw
  line L213 (-487.6237, -2247.1637) -> (-553.1493, -2247.1575)
  arc A243 (-553.6639, -2207.1642) -> (-553.1493, -2247.1575) centre (-553.1474, -2227.1575) ccw
  arc A244 (-916.5761, -1807.1637) -> (-916.5763, -1847.1637) centre (-916.5762, -1827.1637) ccw
  line L214 (-916.5761, -1807.1637) -> (-850.5361, -1807.1642)
  arc A245 (-851.0507, -1847.1575) -> (-850.5361, -1807.1642) centre (-851.0526, -1827.1575) ccw
  line L215 (-851.0507, -1847.1575) -> (-916.5763, -1847.1637)
  line L216 (-183.6639, -1807.1642) -> (-117.6239, -1807.1637)
  arc A246 (-117.6237, -1847.1637) -> (-117.6239, -1807.1637) centre (-117.6238, -1827.1637) ccw
  line L217 (-117.6237, -1847.1637) -> (-183.1493, -1847.1575)
  arc A247 (-183.6639, -1807.1642) -> (-183.1493, -1847.1575) centre (-183.1474, -1827.1575) ccw
  line L218 (-553.6639, -1407.1642) -> (-487.6239, -1407.1637)
  arc A248 (-487.6237, -1447.1637) -> (-487.6239, -1407.1637) centre (-487.6238, -1427.1637) ccw
  line L219 (-487.6237, -1447.1637) -> (-553.1493, -1447.1575)
  arc A249 (-553.6639, -1407.1642) -> (-553.1493, -1447.1575) centre (-553.1474, -1427.1575) ccw
  line L220 (-916.5761, -207.1637) -> (-850.5361, -207.1642)
  arc A250 (-851.0507, -247.1575) -> (-850.5361, -207.1642) centre (-851.0526, -227.1575) ccw
  line L221 (-851.0507, -247.1575) -> (-916.5763, -247.1637)
  arc A251 (-916.5761, -207.1637) -> (-916.5763, -247.1637) centre (-916.5762, -227.1637) ccw
  line L222 (-183.6639, -207.1642) -> (-117.6239, -207.1637)
  arc A252 (-117.6237, -247.1637) -> (-117.6239, -207.1637) centre (-117.6238, -227.1637) ccw
  line L223 (-117.6237, -247.1637) -> (-183.1493, -247.1575)
  arc A253 (-183.6639, -207.1642) -> (-183.1493, -247.1575) centre (-183.1474, -227.1575) ccw
  line L224 (-666.0507, -647.1575) -> (-731.5763, -647.1637)
  arc A254 (-731.5761, -607.1637) -> (-731.5763, -647.1637) centre (-731.5762, -627.1637) ccw
  line L225 (-731.5761, -607.1637) -> (-665.5361, -607.1642)
  arc A255 (-666.0507, -647.1575) -> (-665.5361, -607.1642) centre (-666.0526, -627.1575) ccw
  arc A256 (-916.5761, -1007.1637) -> (-916.5763, -1047.1637) centre (-916.5762, -1027.1637) ccw
  line L226 (-916.5761, -1007.1637) -> (-850.5361, -1007.1642)
  arc A257 (-851.0507, -1047.1575) -> (-850.5361, -1007.1642) centre (-851.0526, -1027.1575) ccw
  line L227 (-851.0507, -1047.1575) -> (-916.5763, -1047.1637)
  line L228 (-183.6639, -1007.1642) -> (-117.6239, -1007.1637)
  arc A258 (-117.6237, -1047.1637) -> (-117.6239, -1007.1637) centre (-117.6238, -1027.1637) ccw
  line L229 (-117.6237, -1047.1637) -> (-183.1493, -1047.1575)
  arc A259 (-183.6639, -1007.1642) -> (-183.1493, -1047.1575) centre (-183.1474, -1027.1575) ccw
  line L230 (-666.0507, -1047.1575) -> (-731.5763, -1047.1637)
  arc A260 (-731.5761, -1007.1637) -> (-731.5763, -1047.1637) centre (-731.5762, -1027.1637) ccw
  line L231 (-731.5761, -1007.1637) -> (-665.5361, -1007.1642)
  arc A261 (-666.0507, -1047.1575) -> (-665.5361, -1007.1642) centre (-666.0526, -1027.1575) ccw
  arc A262 (-916.5761, -607.1637) -> (-916.5763, -647.1637) centre (-916.5762, -627.1637) ccw
  line L232 (-916.5761, -607.1637) -> (-850.5361, -607.1642)
  arc A263 (-851.0507, -647.1575) -> (-850.5361, -607.1642) centre (-851.0526, -627.1575) ccw
  line L233 (-851.0507, -647.1575) -> (-916.5763, -647.1637)
  line L234 (-183.6639, -607.1642) -> (-117.6239, -607.1637)
  arc A264 (-117.6237, -647.1637) -> (-117.6239, -607.1637) centre (-117.6238, -627.1637) ccw
  line L235 (-117.6237, -647.1637) -> (-183.1493, -647.1575)
  arc A265 (-183.6639, -607.1642) -> (-183.1493, -647.1575) centre (-183.1474, -627.1575) ccw
  arc A266 (-731.5761, -207.1637) -> (-731.5763, -247.1637) centre (-731.5762, -227.1637) ccw
  line L236 (-731.5761, -207.1637) -> (-665.5361, -207.1642)
  arc A267 (-666.0507, -247.1575) -> (-665.5361, -207.1642) centre (-666.0526, -227.1575) ccw
  line L237 (-666.0507, -247.1575) -> (-731.5763, -247.1637)
  line L238 (-368.6639, -1407.1642) -> (-302.6239, -1407.1637)
  arc A268 (-302.6237, -1447.1637) -> (-302.6239, -1407.1637) centre (-302.6238, -1427.1637) ccw
  line L239 (-302.6237, -1447.1637) -> (-368.1493, -1447.1575)
  arc A269 (-368.6639, -1407.1642) -> (-368.1493, -1447.1575) centre (-368.1474, -1427.1575) ccw
  line L240 (-1036.0507, -1447.1575) -> (-1101.5763, -1447.1637)
  arc A270 (-1101.5761, -1407.1637) -> (-1101.5763, -1447.1637) centre (-1101.5762, -1427.1637) ccw
  line L241 (-1101.5761, -1407.1637) -> (-1035.5361, -1407.1642)
  arc A271 (-1036.0507, -1447.1575) -> (-1035.5361, -1407.1642) centre (-1036.0526, -1427.1575) ccw
  line L242 (-666.0507, -1847.1575) -> (-731.5763, -1847.1637)
  arc A272 (-731.5761, -1807.1637) -> (-731.5763, -1847.1637) centre (-731.5762, -1827.1637) ccw
  line L243 (-731.5761, -1807.1637) -> (-665.5361, -1807.1642)
  arc A273 (-666.0507, -1847.1575) -> (-665.5361, -1807.1642) centre (-666.0526, -1827.1575) ccw
  line L244 (-368.6639, -2207.1642) -> (-302.6239, -2207.1637)
  arc A274 (-302.6237, -2247.1637) -> (-302.6239, -2207.1637) centre (-302.6238, -2227.1637) ccw
  line L245 (-302.6237, -2247.1637) -> (-368.1493, -2247.1575)
  arc A275 (-368.6639, -2207.1642) -> (-368.1493, -2247.1575) centre (-368.1474, -2227.1575) ccw
  line L246 (-1036.0507, -2247.1575) -> (-1101.5763, -2247.1637)
  arc A276 (-1101.5761, -2207.1637) -> (-1101.5763, -2247.1637) centre (-1101.5762, -2227.1637) ccw
  line L247 (-1101.5761, -2207.1637) -> (-1035.5361, -2207.1642)
  arc A277 (-1036.0507, -2247.1575) -> (-1035.5361, -2207.1642) centre (-1036.0526, -2227.1575) ccw
  circle A278 centre (-171.45, -965.2) radius 9.525
  circle A279 centre (-171.45, -1778) radius 9.525
  circle A280 centre (-171.45, -2286) radius 9.525
  dimension "d111" = 25.4
  dimension "d112" = 6.35
  dimension "d113" = 171.45
  dimension "d114" = 254
  dimension "d115" = 203.2
  dimension "d116" = 6.35
  dimension "d117" = 165.1
  dimension "d118" = 19.05
  dimension "d119" = 965.2
  dimension "d120" = 19.05
  dimension "d121" = 19.05
  dimension "d122" = 1778
  dimension "d123" = 19.05
  dimension "d124" = 2286
  constraint horizontal L172
  constraint tangent L172 A203
  constraint vertical L173
  constraint vertical L174
  constraint tangent A203 L174
  constraint vertical L175
  constraint tangent L172 A204
  constraint tangent L175 A204
  constraint coincident L173 A205.centre
  constraint coincident L173 A278.centre
  constraint coincident L173 A279.centre
  constraint coincident L173 A280.centre
  measures "d111" distance of L168.start L172
  measures "d112" diameter of A203
  measures "d113" distance of L168.start L173
  measures "d114" distance of L168.start L174
  measures "d115" distance of L168.end L175
  measures "d116" diameter of A204
  measures "d117" vertical distance of L168.start A205.centre
  measures "d118" diameter of A205
  measures "d119" vertical distance of L168.start A278.centre
  measures "d120" diameter of A278
  measures "d121" diameter of A279
  measures "d122" vertical distance of L168.start A279.centre
  measures "d123" diameter of A280
  measures "d124" vertical distance of L168.start A280.centre
sketch "Modifications" plane through (0, 0, 19.05) normal (0, 0, 1) x (-1, 0, 0) in component "SpoilBoard"
  line L0 (92.0292, -25.4) -> (-1313.4809, -25.4) construction
  line L1 (-165.1, -2546.2645) -> (-165.1, 117.8725) construction
  line L2 (-254, 110.3437) -> (-254, -155.8083) construction
  circle A0 centre (-257.175, -22.225) radius 3.175
  line L3 (-1016, -79.197) -> (-1016, 74.1427) construction
  circle A1 centre (-1019.175, -22.225) radius 3.175
  circle A2 centre (-165.1, -165.1) radius 9.525
  circle A3 centre (-165.1, -965.2) radius 9.525
  circle A4 centre (-165.1, -1765.3) radius 9.525
  circle A5 centre (-165.1, -2286) radius 9.525
  point P0 (-1219.2, 0)
  dimension "d125" = 165.1
  dimension "d126" = 25.4
  dimension "d127" = 254
  dimension "d128" = 6.35
  dimension "d129" = 203.2
  dimension "d130" = 6.35
  dimension "d131" = 19.05
  dimension "d132" = 165.1
  dimension "d133" = 19.05
  dimension "d134" = 965.2
  dimension "d135" = 19.05
  dimension "d136" = 1765.3
  dimension "d137" = 19.05
  dimension "d138" = 2286
  constraint horizontal L0
  constraint vertical L1
  constraint vertical L2
  constraint tangent L2 A0
  constraint tangent L0 A0
  constraint vertical L3
  constraint tangent L3 A1
  constraint tangent L0 A1
  constraint coincident L1 A2.centre
  constraint coincident L1 A3.centre
  constraint coincident L1 A4.centre
  constraint coincident L1 A5.centre
  measures "d125" horizontal distance of origin L1.end
  measures "d126" vertical distance of origin L0.start
  measures "d127" horizontal distance of origin L2.start
  measures "d128" diameter of A0
  measures "d129" horizontal distance of L3.end P0
  measures "d130" diameter of A1
  measures "d131" diameter of A2
  measures "d132" vertical distance of origin A2.centre
  measures "d133" diameter of A3
  measures "d134" vertical distance of origin A3.centre
  measures "d135" diameter of A4
  measures "d136" vertical distance of origin A4.centre
  measures "d137" diameter of A5
  measures "d138" vertical distance of origin A5.centre
extrude "Extrude6" [suppressed] in component "SpoilBoard"
extrude "Extrude7" [suppressed] in component "SpoilBoard"